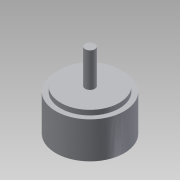
# Autodesk Inventor part: Vishay-157
Saved by Autodesk Inventor 2016 (Build 200138000, 138)
## iProperties
Created: 2016-01-27
Part Number: Vishay-157
Material: Aluminium 6061
Document SubType Name: Modeling
Designer: sd
Mass: 14.0563 g
Surface Area: 17.0871 cm^2
Volume: 5.18681 cm^3
Density: 2.71 g/cm^3
Appearance: Aluminium - Plat
Author: sd
Autodesk Inventor part; units mm, degrees
ref_plane "YZ Plane" through (0, 0, 0) normal (1, 0, 0) x (0, 1, 0)
ref_plane "XZ Plane" through (0, 0, 0) normal (0, 1, 0) x (-1, 0, 0)
ref_plane "XY Plane" through (0, 0, 0) normal (0, 0, 1) x (1, 0, 0)
sketch "Esquisse1" plane through (0, 0, 0) normal (0, 0, 1) x (1, 0, 0)
  circle A0 centre (0, 0) radius 11.1
  dimension "d0" = 22.2
  constraints: 1 centre point, 1 coincident
  measures "d0" diameter of A0
extrude "Extrusion1" add sketch "Esquisse1" along normal blind 13.4
sketch "Esquisse2" plane through (0, 0, 13.4) normal (0, 0, 1) x (1, 0, 0)
  circle A0 centre (0, 0) radius 11.1 projected
  circle A1 centre (0, 0) radius 9.525
  dimension "d3" = 19.05
  constraints: 1 centre point, 1 coincident
  measures "d3" diameter of A1
extrude "Extrusion2" cut sketch "Esquisse2" against normal blind 1.57
sketch "Esquisse4" plane through (0, 0, 13.4) normal (0, 0, 1) x (1, 0, 0)
  circle A0 centre (0, 0) radius 9.525 projected
  circle A1 centre (0, 0) radius 1.585
  dimension "d7" = 3.17
  constraints: 1 centre point, 1 coincident
  measures "d7" diameter of A1
extrude "Extrusion3" add sketch "Esquisse4" along normal blind 11.13 contours A1
